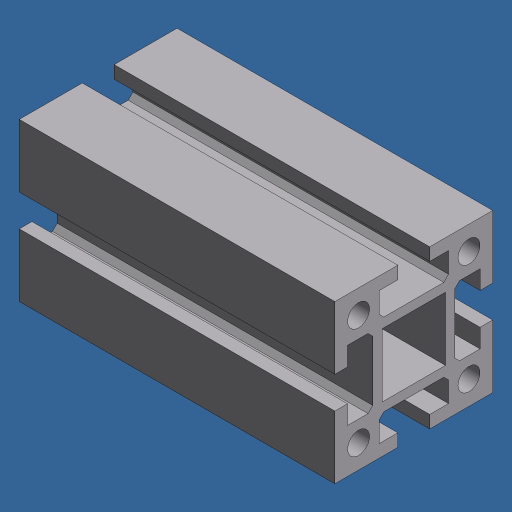
# Autodesk Inventor part: BAR, EXTRUDED ALUM, 50MMX50MM, MK, 2000 SERIES
Saved by Autodesk Inventor 2024.3 (Build 283343000, 343)
## iProperties
Category: _
Manager: _
Created: 2023-11-08
Part Number: BAR, EXTRUDED ALUM, 50MMX50MM, MK, 2000 SERIES
Document SubType Name: Modeling
Designer: -
Manufacturer: Standard
Standards Organization: Custom
Density: 2.71 g/cm^3
Material: Aluminum, 6061-T6
Mass: 294.157 g
Surface Area: 574.244 cm^2
Volume: 108.545 cm^3
Checked By: 00
Engr Approved By: R
User Status: Work In Process
Description: BAR, EXTRUDED ALUM, 50MMX50MM, MK, 2000 SERIES
Mfg Approved By: Stephen.Oerton
Appearance: Aluminum (Flat)
ILogicPurgeVersion: 2.2.20.20
OnSaveVersion: 2.2.20.20
CN_MASS: 0.29
CN_SERVICEABLE: _
CL_runCount: 0
FIRST_DESCRIPTION: _
SECOND_DESCRIPTION: _
THIRD_DESCRIPTION: _
ModelCat: Uncategorized
Author: -
Subject: _
Revision Number: A
Keywords: -
Autodesk Inventor part; units mm, degrees
ref_plane "YZ Plane" through (0, 0, 0) normal (1, 0, 0) x (0, 1, 0)
ref_plane "XZ Plane" through (0, 0, 0) normal (0, 1, 0) x (-1, 0, 0)
ref_plane "XY Plane" through (0, 0, 0) normal (0, 0, 1) x (1, 0, 0)
sketch "Skizze_1" plane through (0, 0, 0) normal (1, 0, 0) x (0, 0, 1)
  line L0 (0, 0) -> (-19.95, 0)
  line L1 (-19.95, 0) -> (-19.95, -4)
  line L2 (-19.95, -4) -> (-14, -4)
  line L3 (-14, -4) -> (-14, -10.5)
  line L4 (-14, -10.5) -> (-15.5, -12)
  line L5 (-15.5, -12) -> (-34.5, -12)
  line L6 (-34.5, -12) -> (-36, -10.5)
  line L7 (-36, -10.5) -> (-36, -4)
  line L8 (-36, -4) -> (-30.05, -4)
  line L9 (-30.05, -4) -> (-30.05, 0)
  line L10 (-30.05, 0) -> (-50, 0)
  line L11 (-50, 0) -> (-50, -19.95)
  line L12 (-50, -19.95) -> (-46, -19.95)
  line L13 (-46, -19.95) -> (-46, -14)
  line L14 (-46, -14) -> (-39.5, -14)
  line L15 (-39.5, -14) -> (-38, -15.5)
  line L16 (-38, -15.5) -> (-38, -34.5)
  line L17 (-38, -34.5) -> (-39.5, -36)
  line L18 (-39.5, -36) -> (-46, -36)
  line L19 (-46, -36) -> (-46, -30.05)
  line L20 (-46, -30.05) -> (-50, -30.05)
  line L21 (-50, -30.05) -> (-50, -50)
  line L22 (-50, -50) -> (-30.05, -50)
  line L23 (-30.05, -50) -> (-30.05, -46)
  line L24 (-30.05, -46) -> (-36, -46)
  line L25 (-36, -46) -> (-36, -39.5)
  line L26 (-36, -39.5) -> (-34.5, -38)
  line L27 (-34.5, -38) -> (-15.5, -38)
  line L28 (-15.5, -38) -> (-14, -39.5)
  line L29 (-14, -39.5) -> (-14, -46)
  line L30 (-14, -46) -> (-19.95, -46)
  line L31 (-19.95, -46) -> (-19.95, -50)
  line L32 (-19.95, -50) -> (0, -50)
  line L33 (0, -50) -> (0, -30.05)
  line L34 (0, -30.05) -> (-4, -30.05)
  line L35 (-4, -30.05) -> (-4, -36)
  line L36 (-4, -36) -> (-10.5, -36)
  line L37 (-10.5, -36) -> (-12, -34.5)
  line L38 (-12, -34.5) -> (-12, -15.5)
  line L39 (-12, -15.5) -> (-10.5, -14)
  line L40 (-10.5, -14) -> (-4, -14)
  line L41 (-4, -14) -> (-4, -19.95)
  line L42 (-4, -19.95) -> (0, -19.95)
  line L43 (0, -19.95) -> (0, 0)
  circle A0 centre (-42.5, -42.5) radius 3.5
  circle A1 centre (-42.5, -7.5) radius 3.5
  line L44 (-14.95, -35.05) -> (-14.95, -14.95)
  line L45 (-14.95, -14.95) -> (-35.05, -14.95)
  line L46 (-35.05, -14.95) -> (-35.05, -35.05)
  line L47 (-35.05, -35.05) -> (-14.95, -35.05)
  circle A2 centre (-7.5, -42.5) radius 3.5
  circle A3 centre (-7.5, -7.5) radius 3.5
  constraints: 96 end point, 4 centre point
extrude "MK, 50MM" add sketch "Skizze_1" along normal blind 100
